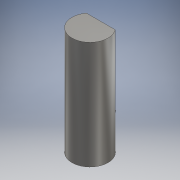
# Autodesk Inventor part: Belt encoder shaft
Saved by Autodesk Inventor 2018 (Build 220112000, 112)
## iProperties
Created: 2017-05-30
Part Number: Belt encoder shaft
Material: Steel
Document SubType Name: Modeling
Designer: M220404
Density: 7.85 g/cm^3
Appearance: Semi-Polished
Author: M220404
Autodesk Inventor part; units mm, degrees
ref_plane "XZ Plane" through (0, 0, 0) normal (0, 1, 0) x (-1, 0, 0)
ref_plane "XY Plane" through (0, 0, 0) normal (0, 0, 1) x (1, 0, 0)
sketch "Sketch1" plane through (0, 0, 0) normal (0, 0, 1) x (1, 0, 0)
  circle A0 centre (0, 0) radius 2.5
  dimension "d0" = 5
  constraints: 1 centre point, 1 coincident
  measures "d0" diameter of A0
extrude "Extrusion1" add sketch "Sketch1" along normal blind 15
ref_plane "Work Plane2" through (-2.5, 0, 0) normal (1, 0, 0) x (0, 1, 0)
sketch "Sketch2" plane through (-2.5, 0, 0) normal (1, 0, 0) x (0, 1, 0)
  line L0 (2.5, 15) -> (-2.5, 15) projected
  line L1 (2.5, 15) -> (-2.5, 15) projected
  line L2 (-2.5, 0) -> (2.5, 0) projected
  line L3 (2.5, 0) -> (2.5, 15) projected
  line L4 (2.5, 15) -> (1.5, 15)
  line L5 (1.5, 15) -> (1.5, 5)
  line L6 (1.5, 5) -> (2.5, 5)
  line L7 (2.5, 5) -> (2.5, 15)
  point P0 (0, 0)
  dimension "d5" = 1
  dimension "d6" = 10
  constraints: 8 end point, 2 parallel, 1 horizontal, 1 perpendicular
  measures "d5" distance of L6.end L5.end
  measures "d6" distance of L5.end L4.end
extrude "Extrusion2" cut sketch "Sketch2" along normal through all
body "Solid1"
